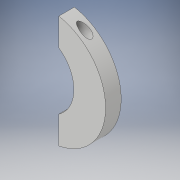
# Autodesk Inventor part: Contrapeso2
Saved by Autodesk Inventor 2019 (Build 230136000, 136)
## iProperties
Created: 2019-06-29
Part Number: Contrapeso2
Material: Generic
Document SubType Name: Modeling
Designer: usuario
Density: 1 g/cm^3
Appearance: Default
Mass: 5.56788 g
Surface Area: 27.2211 cm^2
Volume: 5.56788 cm^3
Author: usuario
Autodesk Inventor part; units mm, degrees
ref_plane "YZ Plane" through (0, 0, 0) normal (1, 0, 0) x (0, 1, 0)
ref_plane "XZ Plane" through (0, 0, 0) normal (0, 1, 0) x (-1, 0, 0)
ref_plane "XY Plane" through (0, 0, 0) normal (0, 0, 1) x (1, 0, 0)
sketch "Sketch1" plane through (0, 0, 0) normal (0, 0, 1) x (1, 0, 0)
  arc A0 (5, -27.0416) -> (5, 27.0416) centre (0, 0) ccw
  line L0 (9.25, 0) -> (0.933, 0)
  line L1 (5, -27.5) -> (5, -13.7954)
  arc A1 (5, -13.7954) -> (5, 13.7954) centre (-4.5, 0) ccw
  arc A2 (5, -27.0416) -> (5, 27.0416) centre (0, 0) ccw
  line L2 (5, 27.5) -> (5, 13.7954)
  line L3 (5, -13.7954) -> (5, -27.5)
  point P0 (-3.7885, 24.6247)
  constraints: 8 end point, 6 point on circle, 3 centre point, 3 vertical, 2 point on line, 1 coincident, 1 horizontal, 1 symmetric about line
extrude "Extrusion1" add sketch "Sketch1" along normal blind 7.5
sketch "Sketch3" plane through (5, -27.0416, 0) normal (-1, 0, 0) x (0, 0, 1)
  line L0 (0, 6.9167) -> (7.5, 6.9167)
  line L1 (0, 0) -> (0, 6.9167)
  line L2 (0, 6.9167) -> (7.5, 6.9167)
  line L3 (7.5, 26.7893) -> (7.5, 0)
  line L4 (7.5, 6.9167) -> (7.5, 0)
  line L5 (7.5, 0) -> (0, 0)
  line L6 (7.5, 0) -> (0, 0)
  circle A0 centre (3.75, 3.963) radius 1
  line L7 (0, 0) -> (0, 53.5786)
  line L8 (0, 53.5786) -> (0, 0)
  line L9 (0, 26.7893) -> (7.5, 26.7893)
  circle A1 centre (3.75, 50.6249) radius 1
  line L10 (0, 53.5786) -> (7.5, 53.5786)
  line L11 (7.5, 53.5786) -> (7.5, 0)
  line L12 (7.5, 54.0833) -> (0.9403, 54.0833)
  line L13 (0, 54.0833) -> (7.5, 54.0833) projected
  circle A2 centre (3.75, 3.963) radius 2
  circle A3 centre (3.75, 50.6249) radius 2
  point P0 (0, 27.0416)
  point P1 (280.32, 51.414)
  dimension "d7" = 2
  dimension "d10" = 4
  dimension "d11" = 4
  constraints: 26 end point, 4 centre point, 2 coincident, 2 collinear, 2 perpendicular, 2 vertical, 1 horizontal, 1 midpoint, 1 point on line
  measures "d7" diameter of A0
  measures "d10" diameter of A2
  measures "d11" diameter of A3
extrude "Extrusion3" cut sketch "Sketch3" against normal blind 25.4 contours A0 | A1
extrude "Extrusion4" cut sketch "Sketch3" against normal blind 17.9375 contours A2 | A3
scale "Scale1" factors (0.5, 0.5, 0.5) then translate (2.5, -6.8977, 3.75) bodies 1
body "Solid1"
